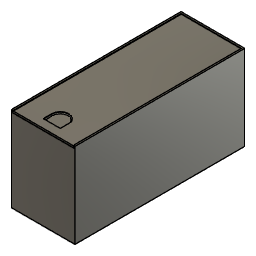
Storage Box (Autodesk Fusion 360 design; units mm, degrees)
Autodesk Fusion 360 part; units mm, degrees
sketch "Sketch1" plane through (0, 0, 0) normal (0, 1, 0) x (1, 0, 0)
  line L0 (0, 0) -> (75, 0)
  line L1 (75, 0) -> (75, -200)
  line L2 (75, -200) -> (0, -200)
  line L3 (0, -200) -> (0, 0)
  line L4 (2, -2) -> (73, -2)
  line L5 (73, -2) -> (73, -198)
  line L6 (73, -198) -> (2, -198)
  line L7 (2, -198) -> (2, -2)
  dimension "d5" = 2
  dimension "d6" = 2
  dimension "d7" = 2
  dimension "d8" = 2
  dimension "d9" = 200
  dimension "d10" = 75
  constraint horizontal L0
  constraint vertical L1
  constraint horizontal L2
  constraint vertical L3
  constraint coincident L0.start L3.end
  constraint horizontal L4
  constraint vertical L5
  constraint horizontal L6
  constraint vertical L7
  measures "d5" distance of L0 L4
  measures "d6" distance of L3 L7
  measures "d7" distance of L1 L5
  measures "d8" distance of L2 L6
  measures "d9" distance of L0.start L2.end
  measures "d10" distance of L0.start L0.end
extrude "Extrude1" add sketch "Sketch1" along normal blind 2 contours L0 L1 L2 L3 | L4 L5 L6 L7 makes body 1
extrude "Extrude2" add sketch "Sketch1" along normal blind 100 bodies 1
sketch "Sketch2" plane through (0, 100, 0) normal (0, 1, 0) x (-1, 0, 0)
  line L0 (-73, 198) -> (-2, 198)
  line L1 (-2, 198) -> (-2, 2)
  line L2 (-2, 2) -> (-73, 2)
  line L3 (-73, 2) -> (-73, 198)
  line L4 (0, 200) -> (-75, 200)
  line L5 (-75, 200) -> (-75, 0)
  line L6 (-75, 0) -> (0, 0)
  line L7 (0, 0) -> (0, 200)
  line L8 (-2, 198) -> (-73, 198)
  line L9 (-73, 198) -> (-73, 200)
  line L10 (-73, 200) -> (-2, 200)
  line L11 (-2, 200) -> (-2, 198)
  line L12 (-1, 1) -> (-74, 1)
  line L13 (-74, 1) -> (-74, 200)
  line L14 (-74, 200) -> (-1, 200)
  line L15 (-1, 200) -> (-1, 1)
  line L16 (-75, 200) -> (-73, 200)
  line L17 (0, 200) -> (-2, 200)
  line L18 (-37.5, 2) -> (-37.5, 0) construction
  constraint horizontal L8
  constraint vertical L9
  constraint horizontal L10
  constraint vertical L11
  constraint coincident L4 L9.end
  constraint coincident L0.end L1.start
  constraint horizontal L12
  constraint vertical L13
  constraint horizontal L14
  constraint vertical L15
  constraint coincident L4 L13.end
  constraint coincident L4.end L5.start
  constraint midpoint L13.end L16
  constraint coincident L4.start L7.end
  constraint midpoint L14.end L17
  constraint coincident L0.start L3.end
  constraint coincident L2 L18.start
  constraint coincident L6 L18.end
  constraint perpendicular L6 L18
  constraint midpoint L12 L18
extrude "Extrude3" cut sketch "Sketch2" against normal blind 2.5 contours L0 L4 L8 L9 L10 L11 L14 bodies 1
extrude "Extrude4" cut sketch "Sketch2" along normal blind 2 from surface at -2.5 contours L1 L2 L3 L4 L9 L11 L12 L13 L14 L15 L16 L17 bodies 1
chamfer "Chamfer1" distance 1 angle 45 3 edges at (1, 99.5, 100.5) (37.5, 99.5, 1) (74, 99.5, 100.5) on bodies 1
sketch "Sketch4" plane through (0, 97.5, 0) normal (0, 1, 0) x (-1, 0, 0)
  line L0 (-2, 198) -> (-2, 2)
  line L1 (-2, 2) -> (-73, 2)
  line L2 (-73, 2) -> (-73, 198)
  line L3 (-1, 200) -> (-74, 200)
  line L4 (-1.2, 200) -> (-73.8, 200)
  line L5 (-73.8, 200) -> (-73.8, 1.2)
  line L6 (-73.8, 1.2) -> (-1.2, 1.2)
  line L7 (-1.2, 1.2) -> (-1.2, 200)
  line L8 (-74, 1) -> (-74, 200)
  line L9 (-1, 1) -> (-74, 1)
  line L10 (-1, 200) -> (-1, 1)
  line L11 (-74, 200) -> (-74, 1)
  line L12 (-74, 1) -> (-1, 1)
  line L13 (-1, 1) -> (-1, 200)
  line L14 (-73, 198) -> (-2, 198)
  dimension "d22" = 0.2
  dimension "d23" = 0.2
  dimension "d24" = 0.2
  constraint horizontal L4
  constraint vertical L5
  constraint horizontal L6
  constraint vertical L7
  constraint coincident L3 L4.start
  measures "d22" distance of L5 L8
  measures "d23" distance of L6 L9
  measures "d24" distance of L7 L10
extrude "Extrude5" add sketch "Sketch4" along normal blind 2 from surface at 50 separate body contours L0 L1 L2 L14 | L3 L4 L5 L6 L7 makes body 2
chamfer "Chamfer2" distance 1 angle 45 3 edges at (1.2, 149.5, 100.6) (37.5, 149.5, 1.2) (73.8, 149.5, 100.6) on bodies 2
sketch "Sketch5" plane through (0, 149.5, 0) normal (0, 1, 0) x (-1, 0, 0)
  line L0 (-72.8, 200) -> (-72.8, 2.2)
  line L1 (-72.8, 2.2) -> (-2.2, 2.2)
  line L2 (-2.2, 2.2) -> (-2.2, 200)
  line L3 (-2.2, 200) -> (-72.8, 200)
  line L4 (-27.5, 190) -> (-47.5, 190)
  line L5 (-47.5, 190) -> (-47.5, 180)
  line L6 (-27.5, 190) -> (-27.5, 180)
  circle A0 centre (-37.5, 180) radius 10
  line L7 (-2.2, 189.9892) -> (-72.8, 189.9892) construction
  line L8 (-37.5, 200) -> (-37.5, 180) construction
  line L9 (-1.2, 200) -> (-73.8, 200) construction
  dimension "d30" = 20
  dimension "d31" = 10
  constraint horizontal L4
  constraint perpendicular L4 L5
  constraint perpendicular L4 L6
  constraint tangent L6 A0
  constraint tangent L5 A0
  constraint coincident L5.end A0
  constraint coincident L6.end A0
  constraint coincident L2 L7.start
  constraint coincident L0 L7.end
  constraint perpendicular L0 L7
  constraint midpoint L3 L8.start
  constraint coincident A0.centre L8
  constraint coincident A0.centre L8.end
  constraint perpendicular L3 L8
  constraint tangent L4 A0
  measures "d30" distance of L4.start L4.end
  measures "d31" distance of L4 L9
extrude "Extrude6" cut sketch "Sketch5" against normal blind 1.5 contours L4 L6 A0 | L4 L5 A0 | A0 bodies 2
fillet "Fillet1" radius 1 3 edges at (27.5, 148, 185) (37.5, 148, 170) (47.5, 148, 185) on bodies 2
copy_body "Body->Comp1" bodies 2 removing the originals makes body 3 in component "Storage Box Lid"
copy_body "Body->Comp2" bodies 1 removing the originals makes body 4 in component "Storage Box"
component "Storage Box Lid" placed x (1, 0, 0) y (0, 1, 0) z (0, 0, 1) at (0, -50, -0.2)
component "Storage Box" placed x (1, 0, 0) y (0, 1, 0) z (0, 0, 1) at (0, 0, 0)
named bodies: "Storage Box", "Storage Box Lid"
